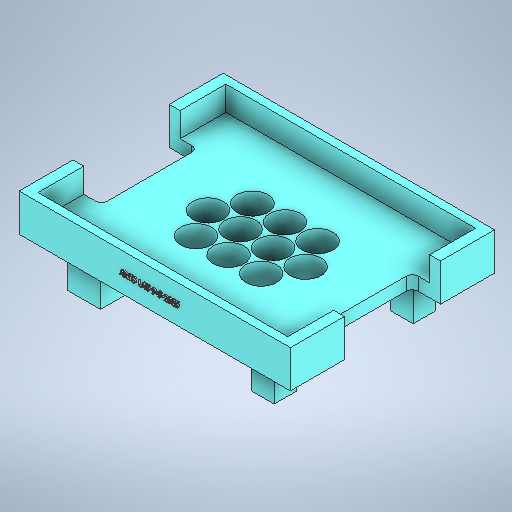
# Autodesk Inventor part: PILLARSCELLCASE18650
Saved by Autodesk Inventor 2025.2 (Build 292293000, 293)
## iProperties
Created: 2024-11-21
Part Number: PILLARSCELLCASE18650
Material: Generic
Document SubType Name: Modeling
Designer: cbast
Density: 1 g/cm^3
Appearance: Default
Mass: 190.937 g
Surface Area: 666.623 cm^2
Volume: 190.937 cm^3
Author: cbast
## iProperties of the stored document BatteryCasev1_3DPrint.ipt
Created: 2025-01-30
Part Number: BatteryCasev1_3DPrint
Material: Generic
Document SubType Name: Modeling
Designer: cbast
Density: 1 g/cm^3
Appearance: Default
Author: cbast
Autodesk Inventor part; units mm, degrees
ref_plane "YZ Plane" through (0, 0, 0) normal (1, 0, 0) x (0, 1, 0)
ref_plane "XZ Plane" through (0, 0, 0) normal (0, 1, 0) x (-1, 0, 0)
ref_plane "XY Plane" through (0, 0, 0) normal (0, 0, 1) x (1, 0, 0)
sketch "Sketch1" plane through (0, 0, 0) normal (0, 1, 0) x (-1, 0, 0)
  circle A0 centre (0, 0) radius 9.5
  circle A1 centre (20, 0) radius 9.5
  circle A2 centre (-20, 0) radius 9.5
  circle A3 centre (-10, 17.3205) radius 9.5
  circle A4 centre (10, 17.3205) radius 9.5
  circle A5 centre (30, 17.3205) radius 9.5
  circle A6 centre (10, -17.3205) radius 9.5
  circle A7 centre (30, -17.3205) radius 9.5
  circle A8 centre (-10, -17.3205) radius 9.5
  circle A9 centre (40, 0) radius 9.5
  line L0 (0, 0) -> (-32.9562, 0) construction
  line L1 (-32.9562, 0) -> (61.076, 0) construction
  circle A10 centre (0, 0) radius 10.5 construction
  circle A11 centre (-20, 0) radius 10.5 construction
  circle A12 centre (-10, -17.3205) radius 10.5 construction
  circle A13 centre (10, -17.3205) radius 10.5 construction
  circle A14 centre (30, -17.3205) radius 10.5 construction
  circle A15 centre (40, 0) radius 10.5 construction
  circle A16 centre (20, 0) radius 10.5 construction
  circle A17 centre (30, 17.3205) radius 10.5 construction
  circle A18 centre (10, 17.3205) radius 10.5 construction
  circle A19 centre (-10, 17.3205) radius 10.5 construction
  circle A20 centre (40, 0) radius 11.5 construction
  circle A21 centre (30, -17.3205) radius 11.5 construction
  circle A22 centre (10, -17.3205) radius 11.5 construction
  circle A23 centre (-10, -17.3205) radius 11.5 construction
  circle A24 centre (-20, 0) radius 11.5 construction
  circle A25 centre (-10, 17.3205) radius 11.5 construction
  circle A26 centre (10, 17.3205) radius 11.5 construction
  circle A27 centre (30, 17.3205) radius 11.5 construction
  circle A28 centre (0, 0) radius 11.5 construction
  circle A29 centre (20, 0) radius 11.5 construction
  arc A30 (39.9181, -11.4997) -> (39.9181, 11.4997) centre (39.9181, 0) ccw
  arc A31 (39.9181, 11.4997) -> (20, 22.9994) centre (30, 17.3205) ccw
  arc A32 (20, 22.9994) -> (0, 22.9994) centre (10, 17.3205) ccw
  arc A33 (0, 22.9994) -> (-19.9181, 11.4997) centre (-10, 17.3205) ccw
  arc A34 (-19.9181, 11.4997) -> (-19.9181, -11.4997) centre (-20, 0) ccw
  arc A35 (-19.9181, -11.4997) -> (0, -22.9994) centre (-10, -17.3205) ccw
  arc A36 (0, -22.9994) -> (20, -22.9994) centre (10, -17.3205) ccw
  arc A37 (20, -22.9994) -> (39.9181, -11.4997) centre (30, -17.3205) ccw
  point P0 (28.893, 7.4235)
  dimension "d0" = 19
  dimension "d2" = 19
  dimension "d4" = 19
  dimension "d6" = 19
  dimension "d8" = 19
  dimension "d10" = 19
  dimension "d11" = 19
  dimension "d13" = 19
  dimension "d14" = 19
  dimension "d53" = 19
  dimension "d91" = 1
  dimension "d144" = 21
  dimension "d145" = 21
  dimension "d146" = 21
  dimension "d147" = 21
  dimension "d148" = 21
  dimension "d149" = 21
  dimension "d150" = 21
  dimension "d151" = 21
  dimension "d152" = 21
  dimension "d153" = 21
  dimension "d154" = 23
  dimension "d155" = 23
  dimension "d156" = 23
  dimension "d157" = 23
  dimension "d158" = 23
  dimension "d159" = 23
  dimension "d160" = 23
  dimension "d161" = 23
  dimension "d162" = 23
  dimension "d163" = 23
  constraints: 38 centre point, 32 point on circle, 22 coincident, 16 tangent, 9 concentric, 4 end point, 2 point on line, 1 horizontal
  measures "d0" diameter of A0
  measures "d2" diameter of A1
  measures "d4" diameter of A2
  measures "d6" diameter of A3
  measures "d8" diameter of A4
  measures "d10" diameter of A5
  measures "d11" diameter of A6
  measures "d13" diameter of A7
  measures "d14" diameter of A8
  measures "d53" diameter of A9
  measures "d144" diameter of A10
  measures "d145" diameter of A11
  measures "d146" diameter of A12
  measures "d147" diameter of A13
  measures "d148" diameter of A14
  measures "d149" diameter of A15
  measures "d150" diameter of A16
  measures "d151" diameter of A17
  measures "d152" diameter of A18
  measures "d153" diameter of A19
  measures "d154" diameter of A20
  measures "d155" diameter of A21
  measures "d156" diameter of A22
  measures "d157" diameter of A23
  measures "d158" diameter of A24
  measures "d159" diameter of A25
  measures "d160" diameter of A26
  measures "d161" diameter of A27
  measures "d162" diameter of A28
  measures "d163" diameter of A29
extrude "Extrusion1" add sketch "Sketch1" along normal blind 15
sketch "Sketch4" plane through (0, 15, 0) normal (0, 1, 0) x (1, 0, 0)
  circle A0 centre (-30, 17.3205) radius 9.5 projected
  circle A1 centre (-40, 0) radius 9.5 projected
  circle A2 centre (-40, 0) radius 9.5 projected
  circle A3 centre (10, 17.3205) radius 9.5 projected
  circle A4 centre (-30, 17.3205) radius 9.5 projected
  circle A5 centre (-10, 17.3205) radius 9.5 projected
  circle A6 centre (-30, -17.3205) radius 9.5 projected
  circle A7 centre (-10, -17.3205) radius 9.5 projected
  circle A8 centre (10, -17.3205) radius 9.5 projected
  circle A9 centre (20, 0) radius 9.5 projected
  circle A10 centre (-20, 0) radius 9.5 projected
  circle A11 centre (0, 0) radius 9.5 projected
  line L0 (0, 0) -> (-10, 0) construction
  line L1 (-86.7, 57.7) -> (66.7, 57.7)
  line L2 (66.7, 57.7) -> (66.7, -57.7)
  line L3 (66.7, -57.7) -> (-86.7, -57.7)
  line L4 (-86.7, -57.7) -> (-86.7, 57.7)
  line L5 (-86.7, 57.7) -> (66.7, -57.7) construction
  line L6 (66.7, 57.7) -> (-86.7, -57.7) construction
  arc A12 (0, 22.9994) -> (-20, 22.9994) centre (-10, 17.3205) ccw projected
  arc A13 (19.9181, 11.4997) -> (0, 22.9994) centre (10, 17.3205) ccw projected
  arc A14 (19.9181, -11.4997) -> (19.9181, 11.4997) centre (20, 0) ccw projected
  arc A15 (0, -22.9994) -> (19.9181, -11.4997) centre (10, -17.3205) ccw projected
  arc A16 (-20, -22.9994) -> (0, -22.9994) centre (-10, -17.3205) ccw projected
  arc A17 (-39.9181, -11.4997) -> (-20, -22.9994) centre (-30, -17.3205) ccw projected
  circle A18 centre (-30, 17.3205) radius 11.5 construction
  arc A19 (-39.9181, 11.4997) -> (-39.9181, -11.4997) centre (-39.9181, 0) ccw projected
  arc A20 (-20, 22.9994) -> (-39.9181, 11.4997) centre (-30, 17.3205) ccw projected
  arc A21 (0, 22.9994) -> (-20, 22.9994) centre (-10, 17.3205) ccw
  arc A22 (19.9181, 11.4997) -> (0, 22.9994) centre (10, 17.3205) ccw
  arc A23 (19.9181, -11.4997) -> (19.9181, 11.4997) centre (20, 0) ccw
  arc A24 (0, -22.9994) -> (19.9181, -11.4997) centre (10, -17.3205) ccw
  arc A25 (-20, -22.9994) -> (0, -22.9994) centre (-10, -17.3205) ccw
  arc A26 (-39.9181, -11.4997) -> (-20, -22.9994) centre (-30, -17.3205) ccw
  arc A27 (-39.9181, 11.4997) -> (-39.9181, -11.4997) centre (-39.9181, 0) ccw
  arc A28 (-20, 22.9994) -> (-39.9181, 11.4997) centre (-30, 17.3205) ccw
  line L7 (-10.5, 0) -> (-9.5, 0) construction
  point P0 (-17.0502, -21.4927)
  point P1 (-17.0502, -11.5134)
  point P2 (-17.0502, -8.8009)
  point P3 (-17.0502, 8.8009)
  point P4 (-17.0502, 11.5134)
  point P5 (-17.0502, 21.4927)
  point P6 (-2.0059, 21.4927)
  point P7 (-2.0059, -11.5134)
  point P8 (-2.0059, -8.8009)
  point P9 (-2.0059, 8.8009)
  point P10 (-2.0059, 11.5134)
  point P11 (-2.0059, -21.4927)
  point P12 (-86.7, 0)
  point P13 (66.7, 0)
  dimension "d104" = 153.4
  dimension "d164" = 115.4
  dimension "d233" = 76.7
  dimension "d234" = 76.7
  constraints: 16 end point, 16 point on circle, 8 centre point, 8 concentric, 5 midpoint, 2 horizontal, 2 parallel, 1 perpendicular, 1 point on line, 4 other
  measures "d104" distance of L2.end L3.end
  measures "d164" distance of L1.end L2.end
  measures "d233" distance of point (-86.7, 0) L0.end
  measures "d234" distance of point (66.7, 0) L0.end
extrude "Extrusion7" add sketch "Sketch4" against normal blind 8 contours L1 L2 L3 L4
sketch "Sketch5" plane through (0, 15, 0) normal (0, 1, 0) x (1, 0, 0)
  line L0 (-86.7, -57.7) -> (66.7, -57.7) projected
  line L1 (66.7, -57.7) -> (66.7, 57.7) projected
  line L2 (66.7, 57.7) -> (-86.7, 57.7) projected
  line L3 (-86.7, 57.7) -> (-86.7, -57.7) projected
  circle A0 centre (-40, 0) radius 9.5 projected
  circle A1 centre (10, 17.3205) radius 9.5 projected
  circle A2 centre (-30, 17.3205) radius 9.5 projected
  circle A3 centre (-10, 17.3205) radius 9.5 projected
  circle A4 centre (-30, -17.3205) radius 9.5 projected
  circle A5 centre (-10, -17.3205) radius 9.5 projected
  circle A6 centre (10, -17.3205) radius 9.5 projected
  circle A7 centre (20, 0) radius 9.5 projected
  circle A8 centre (-20, 0) radius 9.5 projected
  circle A9 centre (0, 0) radius 9.5 projected
  line L4 (-86.7, 57.7) -> (66.7, 57.7)
  line L5 (66.7, 57.7) -> (66.7, -57.7)
  line L6 (66.7, -57.7) -> (-86.7, -57.7)
  line L7 (-86.7, -57.7) -> (-86.7, 57.7)
  line L8 (-93.3464, -62.7) -> (73.3464, -62.7)
  line L9 (73.3464, -62.7) -> (73.3464, 62.7)
  line L10 (73.3464, 62.7) -> (-93.3464, 62.7)
  line L11 (-93.3464, 62.7) -> (-93.3464, -62.7)
  line L12 (-93.3464, -62.7) -> (73.3464, 62.7) construction
  line L13 (73.3464, -62.7) -> (-93.3464, 62.7) construction
  point P0 (66.922, -57.45)
  point P1 (-10, 0)
  dimension "d169" = 5
  dimension "d170" = 6.6464
  dimension "d171" = 166.6929
  dimension "d172" = 125.4
  dimension "d221" = 6.6464
  constraints: 20 end point, 4 parallel, 4 point on line, 2 horizontal, 2 midpoint, 2 perpendicular
  measures "d169" distance between parallel lines of L10 L4
  measures "d170" distance between parallel lines of L9 L5
  measures "d171" distance of L9.end L10.end
  measures "d172" distance of L10.end L8.start
  measures "d221" distance between parallel lines of L3 L11
extrude "Extrusion8" add sketch "Sketch5" along normal blind 15 and the other way blind 8 contours L11 L10 L9 L8
sketch "Sketch6" plane through (0, 15, 0) normal (0, 1, 0) x (1, 0, 0)
  line L0 (59.472, 57.1514) -> (59.472, 25.95) construction
  line L1 (59.472, 25.95) -> (66.7, 25.95) construction
  line L2 (-79.472, -57.7) -> (-79.472, -25.95) construction
  line L3 (-79.472, -25.95) -> (-86.7, -25.95) construction
  circle A0 centre (59.472, 25.95) radius 3.615
  circle A1 centre (59.472, -25.95) radius 3.615
  circle A2 centre (-79.472, -25.95) radius 3.615
  circle A3 centre (-79.472, 25.95) radius 3.615
  line L4 (73.3464, -62.7) -> (73.3464, 62.7) projected
  line L5 (73.3464, 62.7) -> (-93.3464, 62.7) projected
  line L6 (-93.3464, 62.7) -> (-93.3464, -62.7) projected
  line L7 (-93.3464, -62.7) -> (73.3464, -62.7) projected
  line L8 (-86.7, -57.7) -> (-86.7, 57.7) projected
  line L9 (-86.7, 57.7) -> (66.7, 57.7) projected
  line L10 (66.7, 57.7) -> (66.7, -57.7) projected
  line L11 (66.7, -57.7) -> (-86.7, -57.7) projected
  line L12 (-86.7, -57.7) -> (66.7, -57.7) projected
  line L13 (66.7, -57.7) -> (66.7, 57.7) projected
  line L14 (66.7, 57.7) -> (-86.7, 57.7) projected
  line L15 (-86.7, 57.7) -> (-86.7, -57.7) projected
  circle A4 centre (-40, 0) radius 9.5 projected
  circle A5 centre (10, 17.3205) radius 9.5 projected
  circle A6 centre (-30, 17.3205) radius 9.5 projected
  circle A7 centre (-10, 17.3205) radius 9.5 projected
  circle A8 centre (-30, -17.3205) radius 9.5 projected
  circle A9 centre (-10, -17.3205) radius 9.5 projected
  circle A10 centre (10, -17.3205) radius 9.5 projected
  circle A11 centre (20, 0) radius 9.5 projected
  circle A12 centre (-20, 0) radius 9.5 projected
  circle A13 centre (0, 0) radius 9.5 projected
  line L16 (-86.7, 57.7) -> (66.7, 57.7)
  line L17 (66.7, 57.7) -> (66.7, -57.7)
  line L18 (66.7, -57.7) -> (-86.7, -57.7)
  line L19 (-86.7, -57.7) -> (-86.7, 57.7)
  dimension "d123" = 7.23
  dimension "d124" = 7.23
  dimension "d125" = 7.23
  dimension "d140" = 7.23
  dimension "d179" = 31.75
  dimension "d180" = 7.228
  dimension "d181" = 7.228
  dimension "d182" = 31.75
  dimension "d183" = 31.75
  dimension "d184" = 7.228
  dimension "d185" = 7.228
  dimension "d186" = 31.75
  constraints: 16 end point, 4 centre point, 2 coincident, 2 parallel, 1 horizontal, 1 perpendicular
  measures "d123" diameter of A0
  measures "d124" diameter of A1
  measures "d125" diameter of A2
  measures "d140" diameter of A3
  measures "d179" distance from line of A3.centre L16
  measures "d180" distance from line of A3.centre L15
  measures "d181" distance from line of A2.centre L8
  measures "d182" distance from line of L2.end L18
  measures "d183" distance from line of L12 A1.centre
  measures "d184" distance from line of L17 A1.centre
  measures "d185" distance from line of L17 L0.end
  measures "d186" distance from line of L16 L0.end
extrude "Extrusion6" cut sketch "Sketch6" against normal through all contours A0 | A1 | A2 | A3
sketch "Sketch7" plane through (-93.3464, 7, 62.7) normal (-1, 0, 0) x (0, 0, 1)
  line L0 (-120.4, 8) -> (-5, 8) projected
  line L1 (0, 0) -> (-125.4, 0) projected
  line L2 (-125.4, 23) -> (0, 23) projected
  line L3 (-92.265, 8) -> (-85.035, 8) projected
  line L4 (-40.365, 8) -> (-33.135, 8) projected
  line L5 (-92.265, 8) -> (-33.135, 8)
  line L6 (-33.135, 8) -> (-33.135, 23)
  line L7 (-33.135, 23) -> (-92.265, 23)
  line L8 (-92.265, 23) -> (-92.265, 8)
  point P0 (-62.7, -7)
  point P1 (-92.265, 23)
  constraints: 8 end point, 2 parallel, 1 horizontal, 1 perpendicular, 1 point on line
extrude "Extrusion9" cut sketch "Sketch7" against normal through all
sketch "Sketch10" plane through (0, 7, 0) normal (0, -1, 0) x (1, 0, 0)
  circle A0 centre (-79.472, 25.95) radius 3.615 projected
  circle A1 centre (59.472, 25.95) radius 3.615 projected
  circle A2 centre (-79.472, -25.95) radius 3.615 projected
  circle A3 centre (59.472, -25.95) radius 3.615 projected
  line L0 (73.3464, -62.7) -> (73.3464, 62.7) projected
  line L1 (73.3464, 62.7) -> (-93.3464, 62.7) projected
  line L2 (-93.3464, 62.7) -> (-93.3464, -62.7) projected
  line L3 (-93.3464, -62.7) -> (73.3464, -62.7) projected
  arc A4 (-39.9181, -11.4997) -> (-20, -22.9994) centre (-30, -17.3205) ccw projected
  arc A5 (-39.9181, 11.4997) -> (-39.9181, -11.4997) centre (-39.9181, 0) ccw projected
  arc A6 (-20, 22.9994) -> (-39.9181, 11.4997) centre (-30, 17.3205) ccw projected
  arc A7 (0, 22.9994) -> (-20, 22.9994) centre (-10, 17.3205) ccw projected
  arc A8 (19.9181, 11.4997) -> (0, 22.9994) centre (10, 17.3205) ccw projected
  arc A9 (19.9181, -11.4997) -> (19.9181, 11.4997) centre (20, 0) ccw projected
  arc A10 (0, -22.9994) -> (19.9181, -11.4997) centre (10, -17.3205) ccw projected
  arc A11 (-20, -22.9994) -> (0, -22.9994) centre (-10, -17.3205) ccw projected
  line L4 (-93.3464, 62.7) -> (-63.3464, 62.7) construction
  line L5 (-93.3464, 62.7) -> (-93.3464, 42.7) construction
  line L6 (-93.3464, 42.7) -> (-63.3464, 42.7) construction
  line L7 (-73.3464, 52.7) -> (-53.3464, 52.7)
  line L8 (-53.3464, 52.7) -> (-53.3464, 32.7)
  line L9 (-53.3464, 32.7) -> (-73.3464, 32.7)
  line L10 (-73.3464, 32.7) -> (-73.3464, 52.7)
  line L11 (-73.3464, 52.7) -> (-53.3464, 32.7) construction
  line L12 (-53.3464, 52.7) -> (-73.3464, 32.7) construction
  line L13 (-70.8464, 50.2) -> (-55.8464, 50.2)
  line L14 (-55.8464, 50.2) -> (-55.8464, 35.2)
  line L15 (-55.8464, 35.2) -> (-70.8464, 35.2)
  line L16 (-70.8464, 35.2) -> (-70.8464, 50.2)
  line L17 (-70.8464, 50.2) -> (-55.8464, 35.2) construction
  line L18 (-55.8464, 50.2) -> (-70.8464, 35.2) construction
  line L19 (-93.3464, 0) -> (73.3464, 0) construction
  line L20 (-73.3464, -52.7) -> (-53.3464, -52.7)
  line L21 (-53.3464, -52.7) -> (-53.3464, -32.7)
  line L22 (-53.3464, -32.7) -> (-73.3464, -32.7)
  line L23 (-73.3464, -32.7) -> (-73.3464, -52.7)
  line L24 (-73.3464, -52.7) -> (-53.3464, -32.7) construction
  line L25 (-53.3464, -52.7) -> (-73.3464, -32.7) construction
  line L26 (-70.8464, -50.2) -> (-55.8464, -50.2)
  line L27 (-55.8464, -50.2) -> (-55.8464, -35.2)
  line L28 (-55.8464, -35.2) -> (-70.8464, -35.2)
  line L29 (-70.8464, -35.2) -> (-70.8464, -50.2)
  line L30 (-70.8464, -50.2) -> (-55.8464, -35.2) construction
  line L31 (-55.8464, -50.2) -> (-70.8464, -35.2) construction
  line L32 (73.3464, 62.7) -> (43.3464, 62.7) construction
  line L33 (43.3464, 62.7) -> (43.3464, 42.7) construction
  line L34 (36.3464, 49.7) -> (50.3464, 49.7)
  line L35 (50.3464, 49.7) -> (50.3464, 35.7)
  line L36 (50.3464, 35.7) -> (36.3464, 35.7)
  line L37 (36.3464, 35.7) -> (36.3464, 49.7)
  line L38 (36.3464, 49.7) -> (50.3464, 35.7) construction
  line L39 (50.3464, 49.7) -> (36.3464, 35.7) construction
  line L40 (36.3464, -49.7) -> (50.3464, -49.7)
  line L41 (50.3464, -49.7) -> (50.3464, -35.7)
  line L42 (50.3464, -35.7) -> (36.3464, -35.7)
  line L43 (36.3464, -35.7) -> (36.3464, -49.7)
  line L44 (36.3464, -49.7) -> (50.3464, -35.7) construction
  line L45 (50.3464, -49.7) -> (36.3464, -35.7) construction
  line L46 (43.3464, -42.7) -> (43.3464, -62.7) construction
  line L47 (43.3464, -42.7) -> (73.3464, -42.7) construction
  line L48 (-63.3464, -42.7) -> (-63.3464, -62.7) construction
  line L49 (-63.3464, -42.7) -> (-93.3464, -42.7) construction
  point P0 (0, 0)
  dimension "d209" = 30
  dimension "d210" = 20
  dimension "d211" = 20
  dimension "d212" = 20
  dimension "d213" = 15
  dimension "d214" = 15
  dimension "d215" = 30
  dimension "d216" = 20
  dimension "d217" = 14
  dimension "d218" = 14
  dimension "d224" = 30
  dimension "d225" = 30
  dimension "d226" = 20
  dimension "d227" = 20
  constraints: 92 end point, 14 symmetric about line, 8 midpoint, 8 point on line, 7 parallel, 6 perpendicular, 4 horizontal
  measures "d209" distance of L1.end L4.end
  measures "d210" distance of L1.end L5.end
  measures "d211" distance of L8.end L9.end
  measures "d212" distance of L7.end L8.end
  measures "d213" distance of L14.end L15.end
  measures "d214" distance of L13.end L14.end
  measures "d215" distance of L0.end L32.end
  measures "d216" distance of L32.end L33.end
  measures "d217" distance of L35.end L36.end
  measures "d218" distance of L34.end L35.end
  measures "d224" distance of L48.start L49.end
  measures "d225" distance of L46.start L47.end
  measures "d226" distance of L46.start L46.end
  measures "d227" distance of L48.start L48.end
extrude "Extrusion11" add sketch "Sketch10" along normal blind 25 contours L7 L8 L9 L10 | L23 L22 L21 L20 | L34 L35 L36 L37 | L43 L42 L41 L40
sketch "Sketch11" plane through (0, 7, 0) normal (0, -1, 0) x (1, 0, 0)
  line L0 (-70.8464, 50.2) -> (-70.8464, 35.2) projected
  line L1 (-70.8464, 35.2) -> (-55.8464, 35.2) projected
  line L2 (-55.8464, 35.2) -> (-55.8464, 50.2) projected
  line L3 (-55.8464, 50.2) -> (-70.8464, 50.2) projected
  line L4 (-70.8464, 50.2) -> (-55.8464, 50.2)
  line L5 (-55.8464, 50.2) -> (-55.8464, 35.2)
  line L6 (-55.8464, 35.2) -> (-70.8464, 35.2)
  line L7 (-70.8464, 35.2) -> (-70.8464, 50.2)
  line L8 (-55.8464, -35.2) -> (-70.8464, -35.2) projected
  line L9 (-70.8464, -35.2) -> (-70.8464, -50.2) projected
  line L10 (-70.8464, -50.2) -> (-55.8464, -50.2) projected
  line L11 (-55.8464, -50.2) -> (-55.8464, -35.2) projected
  line L12 (-70.8464, -35.2) -> (-55.8464, -35.2)
  line L13 (-55.8464, -35.2) -> (-55.8464, -50.2)
  line L14 (-55.8464, -50.2) -> (-70.8464, -50.2)
  line L15 (-70.8464, -50.2) -> (-70.8464, -35.2)
  point P0 (0, 0)
  constraints: 16 end point, 4 parallel, 2 horizontal, 2 perpendicular
extrude "Extrusion12" add sketch "Sketch11" along normal up to surface (12.5 mm away)
sketch "Sketch13" plane through (0, 7, 0) normal (0, -1, 0) x (1, 0, 0)
  line L0 (36.3464, 35.7) -> (36.3464, 49.7) projected
  line L1 (36.3464, 49.7) -> (50.3464, 49.7) projected
  line L2 (50.3464, 49.7) -> (50.3464, 35.7) projected
  line L3 (50.3464, 35.7) -> (36.3464, 35.7) projected
  line L4 (-73.3464, -32.7) -> (-53.3464, -32.7) projected
  line L5 (-53.3464, -32.7) -> (-53.3464, -52.7) projected
  line L6 (-53.3464, -52.7) -> (-73.3464, -52.7) projected
  line L7 (-73.3464, -52.7) -> (-73.3464, -32.7) projected
  line L8 (36.3464, -49.7) -> (36.3464, -35.7) projected
  line L9 (36.3464, -35.7) -> (50.3464, -35.7) projected
  line L10 (50.3464, -35.7) -> (50.3464, -49.7) projected
  line L11 (50.3464, -49.7) -> (36.3464, -49.7) projected
  line L12 (-73.3464, 32.7) -> (-73.3464, 52.7) projected
  line L13 (-73.3464, 52.7) -> (-53.3464, 52.7) projected
  line L14 (-53.3464, 52.7) -> (-53.3464, 32.7) projected
  line L15 (-53.3464, 32.7) -> (-73.3464, 32.7) projected
  circle A0 centre (-79.472, 25.95) radius 3.615 projected
  circle A1 centre (59.472, 25.95) radius 3.615 projected
  circle A2 centre (-79.472, -25.95) radius 3.615 projected
  circle A3 centre (59.472, -25.95) radius 3.615 projected
  line L16 (73.3464, -62.7) -> (73.3464, 62.7) projected
  line L17 (73.3464, 62.7) -> (-93.3464, 62.7) projected
  line L18 (-93.3464, 62.7) -> (-93.3464, -62.7) projected
  line L19 (-93.3464, -62.7) -> (73.3464, -62.7) projected
  arc A4 (-39.9181, -11.4997) -> (-20, -22.9994) centre (-30, -17.3205) ccw projected
  arc A5 (-39.9181, 11.4997) -> (-39.9181, -11.4997) centre (-39.9181, 0) ccw projected
  arc A6 (-20, 22.9994) -> (-39.9181, 11.4997) centre (-30, 17.3205) ccw projected
  arc A7 (0, 22.9994) -> (-20, 22.9994) centre (-10, 17.3205) ccw projected
  arc A8 (19.9181, 11.4997) -> (0, 22.9994) centre (10, 17.3205) ccw projected
  arc A9 (19.9181, -11.4997) -> (19.9181, 11.4997) centre (20, 0) ccw projected
  arc A10 (0, -22.9994) -> (19.9181, -11.4997) centre (10, -17.3205) ccw projected
  arc A11 (-20, -22.9994) -> (0, -22.9994) centre (-10, -17.3205) ccw projected
  line L20 (-93.3464, 29.565) -> (-75.857, 29.565)
  line L21 (-75.857, 29.565) -> (-75.857, -29.565)
  line L22 (-75.857, -29.565) -> (-93.3464, -29.565)
  line L23 (-93.3464, -29.565) -> (-93.3464, 29.565)
  line L24 (-10, 27.2798) -> (-10, -25.95) construction
  line L25 (73.3464, 29.565) -> (55.857, 29.565)
  line L26 (55.857, 29.565) -> (55.857, -29.565)
  line L27 (55.857, -29.565) -> (73.3464, -29.565)
  circle A12 centre (-79.472, -25.95) radius 3.615 projected
  line L28 (-86.7, 29.565) -> (-86.7, 57.7) projected
  line L29 (-86.7, 57.7) -> (66.7, 57.7) projected
  line L30 (66.7, 57.7) -> (66.7, 29.565) projected
  line L31 (66.7, 29.565) -> (73.3464, 29.565) projected
  line L32 (73.3464, -29.565) -> (73.3464, 29.565) projected
  line L33 (66.7, -29.565) -> (73.3464, -29.565) projected
  line L34 (66.7, -29.565) -> (66.7, -57.7) projected
  line L35 (66.7, -57.7) -> (-86.7, -57.7) projected
  line L36 (-86.7, -57.7) -> (-86.7, -29.565) projected
  line L37 (-93.3464, -29.565) -> (-86.7, -29.565) projected
  line L38 (-93.3464, 29.565) -> (-93.3464, -29.565) projected
  line L39 (-93.3464, 29.565) -> (-86.7, 29.565) projected
  circle A13 centre (59.472, -25.95) radius 3.615 projected
  circle A14 centre (-79.472, 25.95) radius 3.615 projected
  circle A15 centre (-40, 0) radius 9.5 projected
  circle A16 centre (10, -17.3205) radius 9.5 projected
  circle A17 centre (-30, -17.3205) radius 9.5 projected
  circle A18 centre (-10, -17.3205) radius 9.5 projected
  circle A19 centre (-30, 17.3205) radius 9.5 projected
  circle A20 centre (-10, 17.3205) radius 9.5 projected
  circle A21 centre (10, 17.3205) radius 9.5 projected
  circle A22 centre (20, 0) radius 9.5 projected
  circle A23 centre (-20, 0) radius 9.5 projected
  circle A24 centre (0, 0) radius 9.5 projected
  circle A25 centre (59.472, 25.95) radius 3.615 projected
  line L40 (-10.5, 0) -> (-9.5, 0) construction
  point P0 (59.472, -29.565)
  point P1 (59.472, 29.565)
  point P2 (55.857, 25.95)
  point P3 (55.857, -25.95)
  point P4 (-79.472, -29.565)
  point P5 (-75.857, -25.95)
  point P6 (-75.857, 25.95)
  point P7 (-79.472, 29.565)
  dimension "d235" = 17.4895
  dimension "d236" = 17.4895
  constraints: 18 end point, 4 symmetric about line, 2 horizontal, 2 horizontal alignment, 2 parallel, 1 perpendicular, 1 point on line, 1 vertical, 2 other
  measures "d235" distance between parallel lines of L21 L18
  measures "d236" distance between parallel lines of L16 L26
extrude "Extrusion14" cut sketch "Sketch13" against normal blind 10 contours L21 A2 L22 L18 L20 A0 | L25 L16 L27 A3 L26 A1
sketch "Sketch14" plane through (-93.3464, 30, 62.7) normal (0, 0, 1) x (1, 0, 0)
  line L0 (62.5613, -9.7018) -> (99.4197, -9.7018) construction
  line L1 (99.4197, -9.7018) -> (99.4197, -9.6147) construction
  line L2 (99.4197, -9.6147) -> (62.5613, -9.6147) construction
  line L3 (62.5613, -9.6147) -> (62.5613, -9.7018) construction
  line L4 (166.6929, 0) -> (166.6929, -23) projected
  line L5 (0, 0) -> (166.6929, 0) projected
  line L6 (0, -23) -> (0, 0) projected
  line L7 (166.6929, -23) -> (0, -23) projected
  line L8 (83.3464, 0) -> (83.3464, -23) construction
  line L9 (0, -11.5) -> (166.6929, -11.5) construction
  line L10 (62.5416, -12.814) -> (63.5691, -9.766)
  line L11 (63.5691, -9.766) -> (64.068, -9.766)
  line L12 (64.068, -9.766) -> (65.0956, -12.814)
  line L13 (65.0956, -12.814) -> (64.6682, -12.814)
  line L14 (64.6682, -12.814) -> (64.3916, -11.9619)
  line L15 (64.3916, -11.9619) -> (63.2282, -11.9619)
  line L16 (63.2282, -11.9619) -> (62.9516, -12.814)
  line L17 (62.9516, -12.814) -> (62.5416, -12.814)
  line L18 (64.2804, -11.6161) -> (63.8087, -10.181)
  line L19 (63.8087, -10.181) -> (63.3394, -11.6161)
  line L20 (63.3394, -11.6161) -> (64.2804, -11.6161)
  line L21 (67.7434, -12.814) -> (67.2173, -12.814)
  line L22 (67.2173, -12.814) -> (66.254, -11.6013)
  line L23 (66.254, -11.6013) -> (65.7896, -11.6013)
  line L24 (65.7896, -11.6013) -> (65.7896, -12.814)
  line L25 (65.7896, -12.814) -> (65.3845, -12.814)
  line L26 (65.3845, -12.814) -> (65.3845, -9.766)
  line L27 (65.3845, -9.766) -> (66.17, -9.766)
  spline S0 degree 2 poles (66.17, -9.766) (66.4318, -9.766) (66.785, -9.8228) (66.9456, -9.9266) knots 0 0 0 1 2 2 2
  spline S1 degree 2 poles (66.9456, -9.9266) (67.1061, -10.0303) (67.2914, -10.3539) (67.2914, -10.5935) knots 0 0 0 1 2 2 2
  spline S2 degree 2 poles (67.2914, -10.5935) (67.2914, -10.9269) (66.9505, -11.379) (66.6591, -11.4876) knots 0 0 0 1 2 2 2
  line L28 (66.6591, -11.4876) -> (67.7434, -12.814)
  spline S3 degree 2 poles (66.869, -10.6256) (66.869, -10.4922) (66.7752, -10.2872) (66.6764, -10.2205) knots 0 0 0 1 2 2 2
  spline S4 degree 2 poles (66.6764, -10.2205) (66.5899, -10.1637) (66.3602, -10.1168) (66.1922, -10.1168) knots 0 0 0 1 2 2 2
  line L29 (66.1922, -10.1168) -> (65.7896, -10.1168)
  line L30 (65.7896, -10.1168) -> (65.7896, -11.2629)
  line L31 (65.7896, -11.2629) -> (66.1453, -11.2629)
  spline S5 degree 2 poles (66.1453, -11.2629) (66.3207, -11.2629) (66.5998, -11.2011) (66.6961, -11.1048) knots 0 0 0 1 2 2 2
  spline S6 degree 2 poles (66.6961, -11.1048) (66.785, -11.0208) (66.869, -10.7837) (66.869, -10.6256) knots 0 0 0 1 2 2 2
  line L32 (68.6968, -12.814) -> (68.6968, -10.1267)
  line L33 (68.6968, -10.1267) -> (67.6742, -10.1267)
  line L34 (67.6742, -10.1267) -> (67.6742, -9.766)
  line L35 (67.6742, -9.766) -> (70.1245, -9.766)
  line L36 (70.1245, -9.766) -> (70.1245, -10.1267)
  line L37 (70.1245, -10.1267) -> (69.1019, -10.1267)
  line L38 (69.1019, -10.1267) -> (69.1019, -12.814)
  line L39 (69.1019, -12.814) -> (68.6968, -12.814)
  spline S7 degree 2 poles (71.2829, -12.8684) (70.952, -12.8684) (70.4876, -12.7301) (70.2826, -12.6313) knots 0 0 0 1 2 2 2
  line L40 (70.2826, -12.6313) -> (70.2826, -12.1224)
  line L41 (70.2826, -12.1224) -> (70.3122, -12.1224)
  spline S8 degree 2 poles (70.3122, -12.1224) (70.5123, -12.3102) (71.0187, -12.5176) (71.2533, -12.5176) knots 0 0 0 1 2 2 2
  spline S9 degree 2 poles (71.2533, -12.5176) (71.5892, -12.5176) (71.9326, -12.2385) (71.9326, -12.0088) knots 0 0 0 1 2 2 2
  spline S10 degree 2 poles (71.9326, -12.0088) (71.9326, -11.826) (71.7522, -11.5988) (71.5571, -11.542) knots 0 0 0 1 2 2 2
  spline S11 degree 2 poles (71.5571, -11.542) (71.4163, -11.5025) (71.1817, -11.4481) (71.0063, -11.4037) knots 0 0 0 1 2 2 2
  spline S12 degree 2 poles (71.0063, -11.4037) (70.8482, -11.3617) (70.5987, -11.2357) (70.5024, -11.1344) knots 0 0 0 1 2 2 2
  spline S13 degree 2 poles (70.5024, -11.1344) (70.4086, -11.0332) (70.3048, -10.7615) (70.3048, -10.5836) knots 0 0 0 1 2 2 2
  spline S14 degree 2 poles (70.3048, -10.5836) (70.3048, -10.2131) (70.8828, -9.7117) (71.3299, -9.7117) knots 0 0 0 1 2 2 2
  spline S15 degree 2 poles (71.3299, -9.7117) (71.5868, -9.7117) (72.0412, -9.813) (72.2364, -9.9093) knots 0 0 0 1 2 2 2
  line L42 (72.2364, -9.9093) -> (72.2364, -10.3934)
  line L43 (72.2364, -10.3934) -> (72.2067, -10.3934)
  spline S16 degree 2 poles (72.2067, -10.3934) (72.061, -10.26) (71.6065, -10.0624) (71.357, -10.0624) knots 0 0 0 1 2 2 2
  spline S17 degree 2 poles (71.357, -10.0624) (71.0755, -10.0624) (70.7272, -10.3267) (70.7272, -10.5416) knots 0 0 0 1 2 2 2
  spline S18 degree 2 poles (70.7272, -10.5416) (70.7272, -10.7343) (70.9322, -10.964) (71.1249, -11.0159) knots 0 0 0 1 2 2 2
  spline S19 degree 2 poles (71.1249, -11.0159) (71.2533, -11.0504) (71.6263, -11.1394) (71.7498, -11.1764) knots 0 0 0 1 2 2 2
  spline S20 degree 2 poles (71.7498, -11.1764) (72.0635, -11.2727) (72.3549, -11.6605) (72.3549, -11.9446) knots 0 0 0 1 2 2 2
  spline S21 degree 2 poles (72.3549, -11.9446) (72.3549, -12.1249) (72.2092, -12.4707) (72.0783, -12.5917) knots 0 0 0 1 2 2 2
  spline S22 degree 2 poles (72.0783, -12.5917) (71.9326, -12.7251) (71.5621, -12.8684) (71.2829, -12.8684) knots 0 0 0 1 2 2 2
  line L44 (75.8426, -12.814) -> (74.0765, -12.814)
  line L45 (74.0765, -12.814) -> (74.0765, -9.766)
  line L46 (74.0765, -9.766) -> (74.4816, -9.766)
  line L47 (74.4816, -9.766) -> (74.4816, -12.4534)
  line L48 (74.4816, -12.4534) -> (75.8426, -12.4534)
  line L49 (75.8426, -12.4534) -> (75.8426, -12.814)
  line L50 (75.8327, -12.814) -> (76.8602, -9.766)
  line L51 (76.8602, -9.766) -> (77.3592, -9.766)
  line L52 (77.3592, -9.766) -> (78.3867, -12.814)
  line L53 (78.3867, -12.814) -> (77.9594, -12.814)
  line L54 (77.9594, -12.814) -> (77.6828, -11.9619)
  line L55 (77.6828, -11.9619) -> (76.5194, -11.9619)
  line L56 (76.5194, -11.9619) -> (76.2427, -12.814)
  line L57 (76.2427, -12.814) -> (75.8327, -12.814)
  line L58 (77.5716, -11.6161) -> (77.0998, -10.181)
  line L59 (77.0998, -10.181) -> (76.6305, -11.6161)
  line L60 (76.6305, -11.6161) -> (77.5716, -11.6161)
  spline S23 degree 2 poles (80.7431, -11.8779) (80.7431, -12.1051) (80.5702, -12.4534) (80.4269, -12.567) knots 0 0 0 1 2 2 2
  spline S24 degree 2 poles (80.4269, -12.567) (80.254, -12.7004) (79.8613, -12.814) (79.5501, -12.814) knots 0 0 0 1 2 2 2
  line L61 (79.5501, -12.814) -> (78.6757, -12.814)
  line L62 (78.6757, -12.814) -> (78.6757, -9.766)
  line L63 (78.6757, -9.766) -> (79.4834, -9.766)
  spline S25 degree 2 poles (79.4834, -9.766) (79.8094, -9.766) (80.1355, -9.808) (80.2837, -9.8895) knots 0 0 0 1 2 2 2
  spline S26 degree 2 poles (80.2837, -9.8895) (80.4492, -9.976) (80.5998, -10.26) (80.5998, -10.4527) knots 0 0 0 1 2 2 2
  spline S27 degree 2 poles (80.5998, -10.4527) (80.5998, -10.6676) (80.3726, -11.0085) (80.1725, -11.1048) knots 0 0 0 1 2 2 2
  line L64 (80.1725, -11.1048) -> (80.1725, -11.1196)
  spline S28 degree 2 poles (80.1725, -11.1196) (80.4442, -11.1937) (80.7431, -11.5864) (80.7431, -11.8779) knots 0 0 0 1 2 2 2
  spline S29 degree 2 poles (80.3207, -11.8952) (80.3207, -11.7223) (80.2219, -11.5) (80.0737, -11.4209) knots 0 0 0 1 2 2 2
  spline S30 degree 2 poles (80.0737, -11.4209) (79.9774, -11.3715) (79.7502, -11.3419) (79.5402, -11.3419) knots 0 0 0 1 2 2 2
  line L65 (79.5402, -11.3419) -> (79.0808, -11.3419)
  line L66 (79.0808, -11.3419) -> (79.0808, -12.4682)
  line L67 (79.0808, -12.4682) -> (79.4093, -12.4682)
  spline S31 degree 2 poles (79.4093, -12.4682) (79.6761, -12.4682) (79.9823, -12.4188) (80.1009, -12.3398) knots 0 0 0 1 2 2 2
  spline S32 degree 2 poles (80.1009, -12.3398) (80.2145, -12.2583) (80.3207, -12.0557) (80.3207, -11.8952) knots 0 0 0 1 2 2 2
  spline S33 degree 2 poles (80.1775, -10.5095) (80.1775, -10.4008) (80.1034, -10.2378) (80.0219, -10.1909) knots 0 0 0 1 2 2 2
  spline S34 degree 2 poles (80.0219, -10.1909) (79.9231, -10.1365) (79.6835, -10.1118) (79.4686, -10.1118) knots 0 0 0 1 2 2 2
  line L68 (79.4686, -10.1118) -> (79.0808, -10.1118)
  line L69 (79.0808, -10.1118) -> (79.0808, -11.0035)
  line L70 (79.0808, -11.0035) -> (79.5402, -11.0035)
  spline S35 degree 2 poles (79.5402, -11.0035) (79.7304, -11.0035) (79.9107, -10.964) (80.007, -10.9022) knots 0 0 0 1 2 2 2
  spline S36 degree 2 poles (80.007, -10.9022) (80.1009, -10.843) (80.1775, -10.6528) (80.1775, -10.5095) knots 0 0 0 1 2 2 2
  spline S37 degree 2 poles (82.2844, -10.7565) (82.2844, -10.5219) (82.4375, -10.1316) (82.5709, -9.9908) knots 0 0 0 1 2 2 2
  spline S38 degree 2 poles (82.5709, -9.9908) (82.6969, -9.855) (83.0649, -9.7043) (83.2526, -9.7043) knots 0 0 0 1 2 2 2
  spline S39 degree 2 poles (83.2526, -9.7043) (83.4626, -9.7043) (83.8035, -9.8451) (83.9294, -9.9785) knots 0 0 0 1 2 2 2
  spline S40 degree 2 poles (83.9294, -9.9785) (84.0875, -10.1464) (84.2604, -10.6898) (84.2604, -11.1073) knots 0 0 0 1 2 2 2
  spline S41 degree 2 poles (84.2604, -11.1073) (84.2604, -11.4852) (84.09, -12.1619) (83.9245, -12.3867) knots 0 0 0 1 2 2 2
  spline S42 degree 2 poles (83.9245, -12.3867) (83.7491, -12.6238) (83.2551, -12.8733) (82.8945, -12.8733) knots 0 0 0 1 2 2 2
  spline S43 degree 2 poles (82.8945, -12.8733) (82.813, -12.8733) (82.6277, -12.856) (82.5487, -12.8313) knots 0 0 0 1 2 2 2
  line L71 (82.5487, -12.8313) -> (82.5487, -12.4386)
  line L72 (82.5487, -12.4386) -> (82.5684, -12.4386)
  spline S44 degree 2 poles (82.5684, -12.4386) (82.6203, -12.4682) (82.8377, -12.5201) (82.9488, -12.5201) knots 0 0 0 1 2 2 2
  spline S45 degree 2 poles (82.9488, -12.5201) (83.349, -12.5201) (83.8059, -11.9915) (83.838, -11.5025) knots 0 0 0 1 2 2 2
  spline S46 degree 2 poles (83.838, -11.5025) (83.675, -11.6136) (83.3786, -11.7149) (83.2032, -11.7149) knots 0 0 0 1 2 2 2
  spline S47 degree 2 poles (83.2032, -11.7149) (83.0353, -11.7149) (82.7562, -11.6408) (82.6154, -11.5346) knots 0 0 0 1 2 2 2
  spline S48 degree 2 poles (82.6154, -11.5346) (82.4524, -11.4086) (82.2844, -11.0257) (82.2844, -10.7565) knots 0 0 0 1 2 2 2
  spline S49 degree 2 poles (83.8479, -11.0159) (83.8479, -10.7071) (83.7343, -10.3168) (83.633, -10.2106) knots 0 0 0 1 2 2 2
  spline S50 degree 2 poles (83.633, -10.2106) (83.5441, -10.1118) (83.3589, -10.0377) (83.2502, -10.0377) knots 0 0 0 1 2 2 2
  spline S51 degree 2 poles (83.2502, -10.0377) (82.9982, -10.0377) (82.6994, -10.3984) (82.6994, -10.7392) knots 0 0 0 1 2 2 2
  spline S52 degree 2 poles (82.6994, -10.7392) (82.6994, -10.9319) (82.7982, -11.1814) (82.9068, -11.2703) knots 0 0 0 1 2 2 2
  spline S53 degree 2 poles (82.9068, -11.2703) (82.9859, -11.3345) (83.181, -11.3765) (83.2946, -11.3765) knots 0 0 0 1 2 2 2
  spline S54 degree 2 poles (83.2946, -11.3765) (83.4255, -11.3765) (83.7269, -11.2851) (83.8405, -11.2085) knots 0 0 0 1 2 2 2
  spline S55 degree 2 poles (83.8405, -11.2085) (83.843, -11.1789) (83.8479, -11.0776) (83.8479, -11.0159) knots 0 0 0 1 2 2 2
  line L73 (85.7721, -11.6655) -> (84.6186, -11.6655)
  line L74 (84.6186, -11.6655) -> (84.6186, -11.295)
  line L75 (84.6186, -11.295) -> (85.7721, -11.295)
  line L76 (85.7721, -11.295) -> (85.7721, -11.6655)
  spline S56 degree 2 poles (86.9997, -10.055) (86.8885, -10.055) (86.6687, -10.1094) (86.5625, -10.1514) knots 0 0 0 1 2 2 2
  spline S57 degree 2 poles (86.5625, -10.1514) (86.4637, -10.1933) (86.3179, -10.2823) (86.2611, -10.3218) knots 0 0 0 1 2 2 2
  line L77 (86.2611, -10.3218) -> (86.2364, -10.3218)
  line L78 (86.2364, -10.3218) -> (86.2364, -9.8895)
  spline S58 degree 2 poles (86.2364, -9.8895) (86.3698, -9.8179) (86.8268, -9.7018) (87.0318, -9.7018) knots 0 0 0 1 2 2 2
  spline S59 degree 2 poles (87.0318, -9.7018) (87.2392, -9.7018) (87.548, -9.7858) (87.674, -9.8747) knots 0 0 0 1 2 2 2
  spline S60 degree 2 poles (87.674, -9.8747) (87.8074, -9.971) (87.9457, -10.2502) (87.9457, -10.4379) knots 0 0 0 1 2 2 2
  spline S61 degree 2 poles (87.9457, -10.4379) (87.9457, -10.6898) (87.6147, -11.0702) (87.3825, -11.1196) knots 0 0 0 1 2 2 2
  line L79 (87.3825, -11.1196) -> (87.3825, -11.1492)
  spline S62 degree 2 poles (87.3825, -11.1492) (87.4788, -11.169) (87.6987, -11.2579) (87.7925, -11.3468) knots 0 0 0 1 2 2 2
  spline S63 degree 2 poles (87.7925, -11.3468) (87.8864, -11.4333) (88.005, -11.7099) (88.005, -11.91) knots 0 0 0 1 2 2 2
  spline S64 degree 2 poles (88.005, -11.91) (88.005, -12.115) (87.8642, -12.4633) (87.7357, -12.5967) knots 0 0 0 1 2 2 2
  spline S65 degree 2 poles (87.7357, -12.5967) (87.6023, -12.735) (87.2244, -12.8783) (86.9848, -12.8783) knots 0 0 0 1 2 2 2
  spline S66 degree 2 poles (86.9848, -12.8783) (86.7551, -12.8783) (86.3056, -12.7671) (86.1524, -12.6905) knots 0 0 0 1 2 2 2
  line L80 (86.1524, -12.6905) -> (86.1524, -12.2583)
  line L81 (86.1524, -12.2583) -> (86.1821, -12.2583)
  spline S67 degree 2 poles (86.1821, -12.2583) (86.3105, -12.3521) (86.7452, -12.525) (86.9601, -12.525) knots 0 0 0 1 2 2 2
  spline S68 degree 2 poles (86.9601, -12.525) (87.0861, -12.525) (87.338, -12.446) (87.422, -12.3546) knots 0 0 0 1 2 2 2
  spline S69 degree 2 poles (87.422, -12.3546) (87.5035, -12.2632) (87.59, -12.0459) (87.59, -11.8804) knots 0 0 0 1 2 2 2
  spline S70 degree 2 poles (87.59, -11.8804) (87.59, -11.7149) (87.4937, -11.5) (87.4072, -11.4382) knots 0 0 0 1 2 2 2
  spline S71 degree 2 poles (87.4072, -11.4382) (87.3208, -11.3765) (87.0861, -11.3296) (86.9478, -11.3296) knots 0 0 0 1 2 2 2
  line L82 (86.9478, -11.3296) -> (86.7749, -11.3296)
  line L83 (86.7749, -11.3296) -> (86.7749, -10.9912)
  line L84 (86.7749, -10.9912) -> (86.9107, -10.9912)
  spline S72 degree 2 poles (86.9107, -10.9912) (87.1849, -10.9912) (87.5307, -10.7293) (87.5307, -10.4799) knots 0 0 0 1 2 2 2
  spline S73 degree 2 poles (87.5307, -10.4799) (87.5307, -10.3638) (87.4418, -10.1983) (87.3702, -10.1489) knots 0 0 0 1 2 2 2
  spline S74 degree 2 poles (87.3702, -10.1489) (87.2936, -10.097) (87.1059, -10.055) (86.9997, -10.055) knots 0 0 0 1 2 2 2
  line L85 (89.5808, -11.6655) -> (88.4273, -11.6655)
  line L86 (88.4273, -11.6655) -> (88.4273, -11.295)
  line L87 (88.4273, -11.295) -> (89.5808, -11.295)
  line L88 (89.5808, -11.295) -> (89.5808, -11.6655)
  line L89 (91.8656, -12.814) -> (89.9859, -12.814)
  line L90 (89.9859, -12.814) -> (89.9859, -12.3818)
  spline S75 degree 2 poles (89.9859, -12.3818) (90.1884, -12.1916) (90.5491, -11.8384) (90.722, -11.6482) knots 0 0 0 1 2 2 2
  spline S76 degree 2 poles (90.722, -11.6482) (91.0702, -11.2653) (91.3247, -10.8059) (91.3247, -10.5614) knots 0 0 0 1 2 2 2
  spline S77 degree 2 poles (91.3247, -10.5614) (91.3247, -10.4329) (91.2456, -10.2403) (91.174, -10.1785) knots 0 0 0 1 2 2 2
  spline S78 degree 2 poles (91.174, -10.1785) (91.1024, -10.1168) (90.9146, -10.055) (90.801, -10.055) knots 0 0 0 1 2 2 2
  spline S79 degree 2 poles (90.801, -10.055) (90.6923, -10.055) (90.47, -10.1094) (90.3688, -10.1514) knots 0 0 0 1 2 2 2
  spline S80 degree 2 poles (90.3688, -10.1514) (90.2823, -10.1859) (90.1218, -10.2847) (90.0724, -10.3193) knots 0 0 0 1 2 2 2
  line L91 (90.0724, -10.3193) -> (90.0501, -10.3193)
  line L92 (90.0501, -10.3193) -> (90.0501, -9.8846)
  spline S81 degree 2 poles (90.0501, -9.8846) (90.1761, -9.8228) (90.6281, -9.7018) (90.8307, -9.7018) knots 0 0 0 1 2 2 2
  spline S82 degree 2 poles (90.8307, -9.7018) (91.258, -9.7018) (91.7396, -10.1538) (91.7396, -10.5391) knots 0 0 0 1 2 2 2
  spline S83 degree 2 poles (91.7396, -10.5391) (91.7396, -10.7195) (91.6556, -11.0208) (91.5815, -11.1492) knots 0 0 0 1 2 2 2
  spline S84 degree 2 poles (91.5815, -11.1492) (91.5074, -11.2826) (91.2925, -11.5444) (91.174, -11.6704) knots 0 0 0 1 2 2 2
  spline S85 degree 2 poles (91.174, -11.6704) (90.9813, -11.8804) (90.5095, -12.3299) (90.3688, -12.4608) knots 0 0 0 1 2 2 2
  line L93 (90.3688, -12.4608) -> (91.8656, -12.4608)
  line L94 (91.8656, -12.4608) -> (91.8656, -12.814)
  spline S86 degree 2 poles (94.1701, -11.29) (94.1701, -12.1101) (93.6934, -12.8783) (93.1969, -12.8783) knots 0 0 0 1 2 2 2
  spline S87 degree 2 poles (93.1969, -12.8783) (92.693, -12.8783) (92.2213, -12.0953) (92.2213, -11.2925) knots 0 0 0 1 2 2 2
  spline S88 degree 2 poles (92.2213, -11.2925) (92.2213, -10.4675) (92.698, -9.7043) (93.1969, -9.7043) knots 0 0 0 1 2 2 2
  spline S89 degree 2 poles (93.1969, -9.7043) (93.6983, -9.7043) (94.1701, -10.4947) (94.1701, -11.29) knots 0 0 0 1 2 2 2
  spline S90 degree 2 poles (93.6465, -12.2188) (93.7057, -12.0681) (93.7552, -11.6037) (93.7552, -11.29) knots 0 0 0 1 2 2 2
  spline S91 degree 2 poles (93.7552, -11.29) (93.7552, -10.9763) (93.7057, -10.5144) (93.644, -10.3588) knots 0 0 0 1 2 2 2
  spline S92 degree 2 poles (93.644, -10.3588) (93.5822, -10.2032) (93.3674, -10.0427) (93.1969, -10.0427) knots 0 0 0 1 2 2 2
  spline S93 degree 2 poles (93.1969, -10.0427) (93.0265, -10.0427) (92.8067, -10.2032) (92.7424, -10.3638) knots 0 0 0 1 2 2 2
  spline S94 degree 2 poles (92.7424, -10.3638) (92.6807, -10.5194) (92.6362, -10.9936) (92.6362, -11.2925) knots 0 0 0 1 2 2 2
  spline S95 degree 2 poles (92.6362, -11.2925) (92.6362, -11.6136) (92.6758, -12.0434) (92.74, -12.2113) knots 0 0 0 1 2 2 2
  spline S96 degree 2 poles (92.74, -12.2113) (92.7993, -12.3694) (93.0191, -12.5399) (93.1969, -12.5399) knots 0 0 0 1 2 2 2
  spline S97 degree 2 poles (93.1969, -12.5399) (93.3649, -12.5399) (93.5847, -12.3793) (93.6465, -12.2188) knots 0 0 0 1 2 2 2
  line L95 (96.4401, -12.814) -> (94.5604, -12.814)
  line L96 (94.5604, -12.814) -> (94.5604, -12.3818)
  spline S98 degree 2 poles (94.5604, -12.3818) (94.7629, -12.1916) (95.1235, -11.8384) (95.2964, -11.6482) knots 0 0 0 1 2 2 2
  spline S99 degree 2 poles (95.2964, -11.6482) (95.6447, -11.2653) (95.8991, -10.8059) (95.8991, -10.5614) knots 0 0 0 1 2 2 2
  spline S100 degree 2 poles (95.8991, -10.5614) (95.8991, -10.4329) (95.8201, -10.2403) (95.7485, -10.1785) knots 0 0 0 1 2 2 2
  spline S101 degree 2 poles (95.7485, -10.1785) (95.6768, -10.1168) (95.4891, -10.055) (95.3755, -10.055) knots 0 0 0 1 2 2 2
  spline S102 degree 2 poles (95.3755, -10.055) (95.2668, -10.055) (95.0445, -10.1094) (94.9432, -10.1514) knots 0 0 0 1 2 2 2
  spline S103 degree 2 poles (94.9432, -10.1514) (94.8568, -10.1859) (94.6962, -10.2847) (94.6468, -10.3193) knots 0 0 0 1 2 2 2
  line L97 (94.6468, -10.3193) -> (94.6246, -10.3193)
  line L98 (94.6246, -10.3193) -> (94.6246, -9.8846)
  spline S104 degree 2 poles (94.6246, -9.8846) (94.7506, -9.8228) (95.2026, -9.7018) (95.4051, -9.7018) knots 0 0 0 1 2 2 2
  spline S105 degree 2 poles (95.4051, -9.7018) (95.8324, -9.7018) (96.3141, -10.1538) (96.3141, -10.5391) knots 0 0 0 1 2 2 2
  spline S106 degree 2 poles (96.3141, -10.5391) (96.3141, -10.7195) (96.2301, -11.0208) (96.156, -11.1492) knots 0 0 0 1 2 2 2
  spline S107 degree 2 poles (96.156, -11.1492) (96.0819, -11.2826) (95.867, -11.5444) (95.7485, -11.6704) knots 0 0 0 1 2 2 2
  spline S108 degree 2 poles (95.7485, -11.6704) (95.5558, -11.8804) (95.084, -12.3299) (94.9432, -12.4608) knots 0 0 0 1 2 2 2
  line L99 (94.9432, -12.4608) -> (96.4401, -12.4608)
  line L100 (96.4401, -12.4608) -> (96.4401, -12.814)
  spline S109 degree 2 poles (98.6952, -11.8458) (98.6952, -12.0656) (98.5544, -12.4411) (98.426, -12.5794) knots 0 0 0 1 2 2 2
  spline S110 degree 2 poles (98.426, -12.5794) (98.2975, -12.7177) (97.9147, -12.8783) (97.6775, -12.8783) knots 0 0 0 1 2 2 2
  spline S111 degree 2 poles (97.6775, -12.8783) (97.4602, -12.8783) (97.0353, -12.7819) (96.8797, -12.7054) knots 0 0 0 1 2 2 2
  line L101 (96.8797, -12.7054) -> (96.8797, -12.2731)
  line L102 (96.8797, -12.2731) -> (96.9094, -12.2731)
  spline S112 degree 2 poles (96.9094, -12.2731) (96.9563, -12.3077) (97.1317, -12.3966) (97.2379, -12.4361) knots 0 0 0 1 2 2 2
  spline S113 degree 2 poles (97.2379, -12.4361) (97.3589, -12.4781) (97.559, -12.525) (97.6849, -12.525) knots 0 0 0 1 2 2 2
  spline S114 degree 2 poles (97.6849, -12.525) (97.8084, -12.525) (98.0406, -12.4361) (98.1246, -12.3398) knots 0 0 0 1 2 2 2
  spline S115 degree 2 poles (98.1246, -12.3398) (98.2012, -12.2484) (98.2802, -12.0063) (98.2802, -11.8433) knots 0 0 0 1 2 2 2
  spline S116 degree 2 poles (98.2802, -11.8433) (98.2802, -11.6803) (98.1913, -11.4728) (98.1073, -11.4037) knots 0 0 0 1 2 2 2
  spline S117 degree 2 poles (98.1073, -11.4037) (98.0209, -11.3271) (97.764, -11.2629) (97.6084, -11.2629) knots 0 0 0 1 2 2 2
  spline S118 degree 2 poles (97.6084, -11.2629) (97.4404, -11.2629) (97.107, -11.3147) (97.0057, -11.337) knots 0 0 0 1 2 2 2
  line L103 (97.0057, -11.337) -> (97.0057, -9.766)
  line L104 (97.0057, -9.766) -> (98.6779, -9.766)
  line L105 (98.6779, -9.766) -> (98.6779, -10.1242)
  line L106 (98.6779, -10.1242) -> (97.3984, -10.1242)
  line L107 (97.3984, -10.1242) -> (97.3984, -10.9368)
  spline S119 degree 2 poles (97.3984, -10.9368) (97.4725, -10.9269) (97.6158, -10.9195) (97.6751, -10.9195) knots 0 0 0 1 2 2 2
  spline S120 degree 2 poles (97.6751, -10.9195) (97.9097, -10.9195) (98.2333, -10.9961) (98.3815, -11.1097) knots 0 0 0 1 2 2 2
  spline S121 degree 2 poles (98.3815, -11.1097) (98.5322, -11.2233) (98.6952, -11.5691) (98.6952, -11.8458) knots 0 0 0 1 2 2 2
  point P0 (93.3464, -30)
  constraints: 4 end point, 4 midpoint, 2 other
extrude "Extrusion15" add sketch "Sketch14" along normal blind 1 contours L10 L11 L12 L13 L14 L15 L16 L17 | L21 L22 L23 L24 L25 L26 L27 S0 S1 S2 L28 | L32 L33 L34 L35 L36 L37 L38 L39 | S7 L40 L41 S8 S9 S10 S11 S12 S13 S14 S15 L42 L43 S16 S17 S18 S19 S20 S21 S22 | L44 L50 L49 | L49 L50 L51 L52 L53 L54 L55 L56 L57 | L44 L45 L46 L47 L48 L49 L50 | S23 S24 L61 L62 L63 S25 S26 S27 L64 S28 | S37 S38 S39 S40 S41 S42 S43 L71 L72 S44 S45 S46 S47 S48 | L73 L74 L75 L76 | S56 S57 L77 L78 S58 S59 S60 S61 L79 S62 S63 S64 S65 S66 L80 L81 S67 S68 S69 S70 S71 L82 L83 L84 S72 S73 S74 | L85 L86 L87 L88 | L89 L90 S75 S76 S77 S78 S79 S80 L91 L92 S81 S82 S83 S84 S85 L93 L94 | S86 S87 S88 S89 | L95 L96 S98 S99 S100 S101 S102 S103 L97 L98 S104 S105 S106 S107 S108 L99 L100 | S109 S110 S111 L101 L102 S112 S113 S114 S115 S116 S117 S118 L103 L104 L105 L106 L107 S119 S120 S121
body "Solid1"
